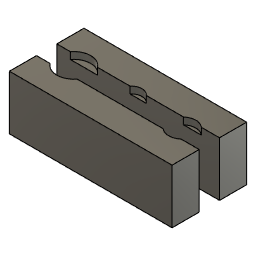
EFM v92 (Autodesk Fusion 360 archive; units mm, degrees)
design "Hub Soft Jaws"
Autodesk Fusion 360 part; units mm, degrees
sketch "Sketch1" plane through (0, 0, 0) normal (0, 1, 0) x (1, 0, 0) in component "Component"
  line L0 (76.2, -9.525) -> (-76.2, -9.525) construction
  line L1 (-76.2, -9.525) -> (-76.2, 9.525) construction
  line L2 (-76.2, 9.525) -> (76.2, 9.525) construction
  line L3 (76.2, 9.525) -> (76.2, -9.525) construction
  line L4 (76.2, -9.525) -> (-76.2, 9.525) construction
  line L5 (-76.2, -9.525) -> (76.2, 9.525) construction
  line L6 (-76.2, 9.525) -> (76.2, 9.525)
  line L7 (76.2, 9.525) -> (76.2, 34.925)
  line L8 (76.2, 34.925) -> (-76.2, 34.925)
  line L9 (-76.2, 34.925) -> (-76.2, 9.525)
  line L10 (-76.2, -9.525) -> (76.2, -9.525)
  line L11 (76.2, -9.525) -> (76.2, -34.925)
  line L12 (76.2, -34.925) -> (-76.2, -34.925)
  line L13 (-76.2, -34.925) -> (-76.2, -9.525)
  circle A0 centre (-50.8, 0) radius 15.875
  line L14 (0, 0) -> (-50.8, 0) construction
  line L15 (0, 0) -> (50.8, 0) construction
  circle A1 centre (50.8, 0) radius 12.7
  circle A2 centre (0, 3.175) radius 9.9187
  dimension "d1" = 152.4
  dimension "d2" = 19.05
  dimension "d3" = 152.4
  dimension "d4" = 25.4
  dimension "d5" = 152.4
  dimension "d6" = 25.4
  dimension "d7" = 31.75
  dimension "d8" = 50.8
  dimension "d9" = 50.8
  dimension "d10" = 25.4
  dimension "d15" = 19.8374
  dimension "d16" = 3.175
  dimension "d17" = 76.2
  constraint horizontal L0
  constraint perpendicular L0 L1
  constraint parallel L0 L2
  constraint parallel L1 L3
  constraint coincident L4 L14.start
  constraint coincident L5 L14.start
  constraint coincident L14.start L15.start
  constraint horizontal L6
  constraint vertical L7
  constraint horizontal L8
  constraint vertical L9
  constraint horizontal L10
  constraint vertical L11
  constraint horizontal L12
  constraint vertical L13
  constraint coincident A0.centre L14.end
  constraint parallel L2 L14
  constraint parallel L14 L15
  constraint coincident L15.end A1.centre
  measures "d1" distance of L1.end L2.end
  measures "d2" distance of L0.end L1.end
  measures "d3" distance of L1.end L2.end
  measures "d4" distance of L1.end L8.end
  measures "d5" distance of L0.end L0.start
  measures "d6" distance of L0.end L12.end
  measures "d7" diameter of A0
  measures "d8" distance of L14.start A0.centre
  measures "d9" distance of L14.start L15.end
  measures "d10" diameter of A1
  measures "d15" diameter of A2
  measures "d16" distance of L14.start A2.centre
  measures "d17" horizontal distance of L1.end A2.centre
extrude "Extrude1" add sketch "Sketch1" against normal blind 50.8 contours L6 L7 L8 L9 A0 A1 A2 | L6 A0 | L10 L11 L12 L13 A0 A1 | L10 A0 | L6 A2 | L10 A1 | L6 A1 picked at (0.481, 11.3734) makes body 1 at (-25.4, -16.9333, 9.525) makes body 2 at (-25.4, -16.9333, -9.525) in component "Component"
extrude "Extrude2" cut sketch "Sketch1" against normal blind 6.35 contours L6 A0 | L10 A0 | L6 A2 | L10 A1 | L6 A1 picked at (0.481, 11.3734) bodies 1 2 in component "Component"
component "Component" placed x (1, 0, 0) y (0, 1, 0) z (0, 0, 1) at (0, 0, 0)
